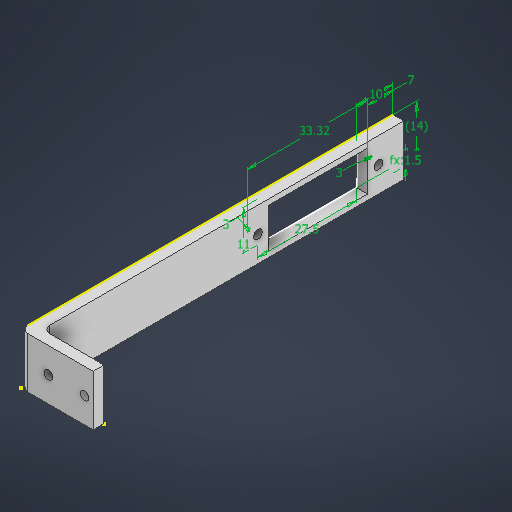
# Autodesk Inventor part: płytka złącza
Saved by Autodesk Inventor 2026.1 (Build 301233020, 233B)
## iProperties
Created: 2026-03-26
Part Number: płytka złącza
Material: Generic
Document SubType Name: Modeling
Designer: Jan
Density: 1 g/cm^3
Appearance: Default
Author: Jan
Autodesk Inventor part; units mm, degrees
ref_plane "YZ Plane" through (0, 0, 0) normal (1, 0, 0) x (0, 1, 0)
ref_plane "XZ Plane" through (0, 0, 0) normal (0, 1, 0) x (-1, 0, 0)
ref_plane "XY Plane" through (0, 0, 0) normal (0, 0, 1) x (1, 0, 0)
sketch "Sketch1" plane through (0, 0, 0) normal (0, 1, 0) x (-1, 0, 0)
  line L0 (0, 0) -> (0, -3)
  line L1 (0, -3) -> (15, -3)
  line L2 (17, -5) -> (17, -102.86)
  line L3 (0, 0) -> (18, 0)
  line L4 (20, -2) -> (20, -102.86)
  line L5 (20, -102.86) -> (17, -102.86)
  arc A0 (17, -5) -> (15, -3) centre (15, -5) ccw
  arc A1 (20, -2) -> (18, 0) centre (18, -2) ccw
  point P0 (17, -3)
  point P1 (20, 0)
  dimension "d0" = 3
  dimension "d1" = 17
  dimension "d2" = 99.86
  dimension "d3" = 20
  dimension "d4" = 2
  constraints: 12 end point, 4 perpendicular, 4 point on circle, 4 point on line, 4 tangent, 2 centre point, 1 equal radius, 1 horizontal, 1 vertical
  measures "d0" distance of L0.start L0.end
  measures "d1" distance of L0.end point (17, -3)
  measures "d2" distance of point (17, -3) L2.end
  measures "d3" distance of L0.start point (20, 0)
  measures "d4" radius of A0
extrude "Extrusion1" add sketch "Sketch1" along normal blind 14
sketch "Sketch2" plane through (0, 0, -3) normal (0, 0, -1) x (-1, 0, 0)
  point P0 (0, 0)
sketch "Sketch3" plane through (0, 0, -3) normal (0, 0, -1) x (-1, 0, 0)
  circle A0 centre (2.3646, 7) radius 1.5
  circle A1 centre (12.3646, 7) radius 1.5
  line L0 (0, 14) -> (15, 14) projected
  line L1 (0, 0) -> (15, 0) projected
  dimension "d7" = 3
  dimension "d8" = 3
  dimension "d9" = 14
  dimension "d10" = 7
  dimension "d11" = 10
  constraints: 2 centre point, 1 horizontal alignment
  measures "d7" diameter of A0
  measures "d8" diameter of A1
  measures "d9" distance between parallel lines of L0 L1
  measures "d10" distance from line of L1 A0.centre
  measures "d11" distance of A1.centre A0.centre
hole "Hole1" at (-2.3646, 7, -3) at (-12.3646, 7, -3) direction (0, 0, 1) diameter 2.459 depth 8.8 tip angle 118 thread size "M3x0.5" class "6H" standard "ISO Metric profile"
sketch "Sketch4" plane through (-20, 0, -102.86) normal (-1, 0, 0) x (0, 0, 1)
  line L0 (10, 12.5) -> (37.5, 12.5)
  line L1 (37.5, 12.5) -> (37.5, 1.5)
  line L2 (37.5, 1.5) -> (10, 1.5)
  line L3 (10, 1.5) -> (10, 12.5)
  line L4 (0, 14) -> (100.86, 14) projected
  line L5 (0, 0) -> (100.86, 0) projected
  line L6 (0, 0) -> (0, 14) projected
  circle A0 centre (7, 7) radius 1.5
  circle A1 centre (40.32, 7) radius 1.5
  point P0 (102.86, 0)
  dimension "d19" = 27.5
  dimension "d20" = 11
  dimension "d21" = 14
  dimension "d22" = 1.5
  dimension "d23" = 10
  dimension "d24" = 3
  dimension "d25" = 3
  dimension "d26" = 33.32
  dimension "d29" = 7
  constraints: 8 end point, 2 centre point, 2 parallel, 1 horizontal, 1 perpendicular
  measures "d19" distance of L1.end L2.end
  measures "d20" distance of L0.end L1.end
  measures "d21" distance between parallel lines of L4 L5
  measures "d22" distance between parallel lines of L2 L5
  measures "d23" distance between parallel lines of L6 L3
  measures "d24" diameter of A0
  measures "d25" diameter of A1
  measures "d26" distance of A1.centre A0.centre
  measures "d29" distance from line of L6 A0.centre
hole "Hole2" at (-20, 7, -62.54) at (-20, 7, -95.86) direction (1, 0, 0) diameter 2.459 depth 8.8 tip angle 118 thread size "M3x0.5" class "6H" standard "ISO Metric profile"
extrude "Extrusion2" cut sketch "Sketch4" against normal blind 14 contours L0 L1 L2 L3
equation "\"d10\" = 0.5 * d9"
equation "\"d22\" = -0.5 * d20 + 0.5 * d21"
body "Solid1"
